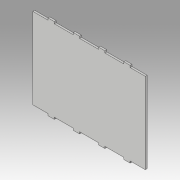
# Autodesk Inventor part: bottom
Saved by Autodesk Inventor 2019.3 (Build 233278000, 278)
## iProperties
Created: 2019-06-26
Part Number: bottom
Material: Generic
Document SubType Name: Modeling
Designer: Dave
Density: 1 g/cm^3
Appearance: Default
Author: Dave
Autodesk Inventor part; units mm, degrees
ref_plane "YZ Plane" through (0, 0, 0) normal (1, 0, 0) x (0, 1, 0)
ref_plane "XZ Plane" through (0, 0, 0) normal (0, 1, 0) x (-1, 0, 0)
ref_plane "XY Plane" through (0, 0, 0) normal (0, 0, 1) x (1, 0, 0)
sketch "Sketch1" plane through (0, 0, 0) normal (0, 0, 1) x (1, 0, 0)
  line L0 (178, 0) -> (178, 128)
  line L1 (0, 128) -> (0, 0)
  line L2 (34, 128) -> (34, 131)
  line L3 (34, 131) -> (24, 131)
  line L4 (24, 131) -> (24, 128)
  line L5 (74, 128) -> (74, 131)
  line L6 (74, 131) -> (64, 131)
  line L7 (64, 131) -> (64, 128)
  line L8 (114, 128) -> (114, 131)
  line L9 (114, 131) -> (104, 131)
  line L10 (104, 131) -> (104, 128)
  line L11 (154, 128) -> (154, 131)
  line L12 (154, 131) -> (144, 131)
  line L13 (144, 131) -> (144, 128)
  line L14 (34, 0) -> (34, -3)
  line L15 (34, -3) -> (24, -3)
  line L16 (24, -3) -> (24, 0)
  line L17 (74, 0) -> (74, -3)
  line L18 (74, -3) -> (64, -3)
  line L19 (64, -3) -> (64, 0)
  line L20 (114, 0) -> (114, -3)
  line L21 (114, -3) -> (104, -3)
  line L22 (104, -3) -> (104, 0)
  line L23 (154, 0) -> (154, -3)
  line L24 (154, -3) -> (144, -3)
  line L25 (144, -3) -> (144, 0)
  line L26 (24, 128) -> (0, 128)
  line L27 (64, 128) -> (34, 128)
  line L28 (104, 128) -> (74, 128)
  line L29 (178, 128) -> (154, 128)
  line L30 (144, 128) -> (114, 128)
  line L31 (0, 0) -> (24, 0)
  line L32 (34, 0) -> (64, 0)
  line L33 (74, 0) -> (104, 0)
  line L34 (114, 0) -> (144, 0)
  line L35 (154, 0) -> (178, 0)
  dimension "d8" = 30
  dimension "d9" = 30
  dimension "d10" = 24
  dimension "d11" = 30
  dimension "d12" = 24
  dimension "d13" = 128
  dimension "d14" = 178
  dimension "d15" = 10
  dimension "d16" = 3
  constraints: 72 end point, 34 parallel, 14 collinear, 14 point on line, 13 equal length, 5 horizontal, 5 perpendicular
  measures "d8" distance of L10.end L5.start
  measures "d9" distance of L7.end L2.start
  measures "d10" distance of L4.end L1.start
  measures "d11" distance of L13.end L8.start
  measures "d12" distance of L0.end L11.start
  measures "d13" distance of L0.start L0.end
  measures "d14" distance between parallel lines of L1 L0
  measures "d15" distance of L2.end L3.end
  measures "d16" distance of L2.start L2.end
extrude "Extrusion1" add sketch "Sketch1" along normal blind 3
body "Solid1"
